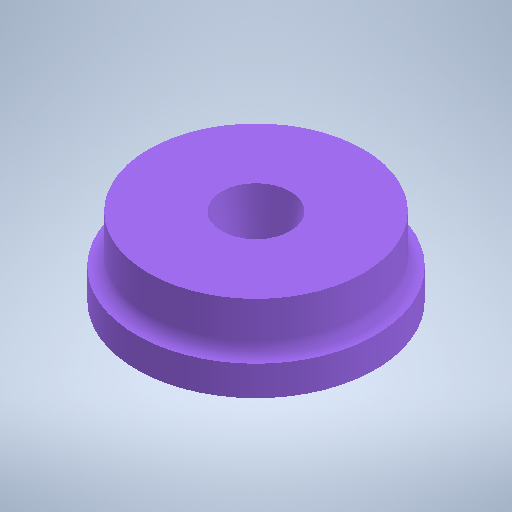
# Autodesk Inventor part: Mitnehmer
Saved by Autodesk Inventor 2025 (Build 290162010, 162A)
## iProperties
Created: 2024-04-30
Part Number: Mitnehmer
Material: Lead
Document SubType Name: Modeling
Designer: ffogue
Density: 11.34 g/cm^3
Appearance: Violet
Author: ffogue
Autodesk Inventor part; units mm, degrees
ref_plane "YZ Plane" through (0, 0, 0) normal (1, 0, 0) x (0, 1, 0)
ref_plane "XY Plane" through (0, 0, 0) normal (0, 0, 1) x (1, 0, 0)
sketch "Skizze1" plane through (0, 0, 0) normal (0, 1, 0) x (-1, 0, 0)
  line L0 (0, 0) -> (18, 0)
  line L1 (18, 0) -> (18, -6)
  arc A0 (18, -6) -> (20, -8) centre (20, -6) ccw
  line L2 (20, -8) -> (20, -13)
  line L3 (20, -13) -> (0, -13)
  line L4 (0, -13) -> (0, 0)
  dimension "d0" = 5
  dimension "d2" = 40
  dimension "d3" = 36
  dimension "d12" = 13
  constraints: 10 end point, 3 perpendicular, 2 point on circle, 1 centre point, 1 horizontal, 1 parallel, 1 tangent, 1 vertical alignment
  measures "d0" distance of L2.start L2.end
  measures "d2" diameter of L2 L4
  measures "d3" diameter of L1 L4
  measures "d12" distance between parallel lines of L0 L3
revolve "Umdrehung1" add sketch "Skizze1" angle 360 about axis through (0, 0, -13) along (0, 0, 1)
ref_plane "Arbeitsebene1" through (0, 0, 0) normal (0, 1, 0) x (-1, 0, 0)
sketch "Skizze2" plane through (0, 0, 0) normal (0, 1, 0) x (-1, 0, 0)
  line L0 (18, 0) -> (-18, 0) projected
  line L1 (20, -13) -> (-20, -13) projected
  line L2 (5.75, 0) -> (3.3056, -11.5)
  line L3 (3.3056, -11.5) -> (10, -11.5)
  line L4 (10, -11.5) -> (10, -12.0712)
  line L5 (10, -12.0712) -> (10, -12.0712)
  line L6 (10, -12.0712) -> (10, -13)
  line L7 (0, 0) -> (0, -13)
  line L8 (5.75, 0) -> (0, 0)
  dimension "d6" = 1.5
  dimension "d7" = 12
  dimension "d8" = 11.5
  dimension "d9" = 20
  constraints: 14 end point, 3 perpendicular, 2 point on line, 1 collinear, 1 horizontal, 1 midpoint, 1 vertical alignment
  measures "d6" distance between parallel lines of L1 L3
  measures "d7" angle of L7 L2
  measures "d8" diameter of L2.start L7
  measures "d9" diameter of L6.end L7
revolve "Umdrehung2" cut sketch "Skizze2" angle 360 about axis through (0, 0, 0) along (0, 0, -1)
